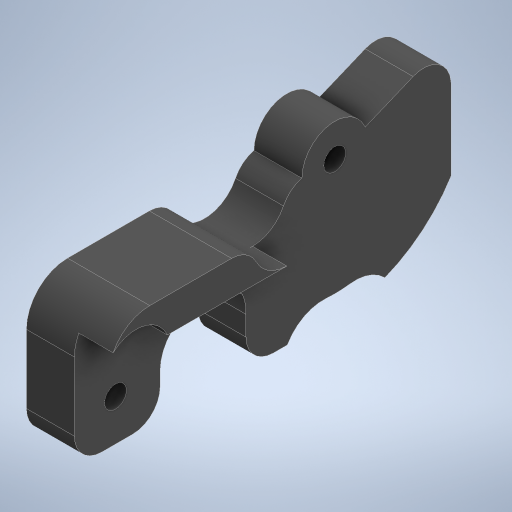
# Autodesk Inventor part: toe_springjoint_cover_under_right
Saved by Autodesk Inventor 2024.1 (Build 281209000, 209)
## iProperties
Created: 2024-02-25
Part Number: toe_springjoint_cover_under_right
Material: 一般
Document SubType Name: Modeling
Designer: hibik
Density: 1 g/cm^3
Appearance: 既定
Author: hibik
Autodesk Inventor part; units mm, degrees
ref_plane "YZ Plane" through (0, 0, 0) normal (1, 0, 0) x (0, 1, 0)
ref_plane "XZ Plane" through (0, 0, 0) normal (0, 1, 0) x (-1, 0, 0)
ref_plane "XY Plane" through (0, 0, 0) normal (0, 0, 1) x (1, 0, 0)
sketch "スケッチ1" plane through (0, 0, 0) normal (1, 0, 0) x (0, 1, 0)
  circle A0 centre (0, 0) radius 6 construction
  circle A1 centre (6, 0) radius 0.8
  line L0 (-14, 0) -> (14, 0)
  circle A2 centre (4.242641, 4.242641) radius 0.8
  circle A3 centre (0, 6) radius 0.8
  circle A4 centre (-4.242641, 4.242641) radius 0.8
  circle A5 centre (-6, 0) radius 0.8
  circle A6 centre (-4.242641, -4.242641) radius 0.8
  circle A7 centre (0, -6) radius 0.8
  circle A8 centre (4.242641, -4.242641) radius 0.8
  circle A9 centre (0, 0) radius 2.4
  line L1 (0, 0) -> (0, 6)
  line L2 (0, 0) -> (2.296101, -5.543277)
  circle A10 centre (0, 0) radius 10
  line L3 (2.296101, -5.543277) -> (3.826834, -9.238795)
  line L4 (0, -9.238795) -> (-10, -9.238795)
  line L5 (-10, -9.238795) -> (-10, 20)
  line L6 (-10, 20) -> (0, 20)
  line L7 (0, 20) -> (0, -9.238795)
  line L8 (0, -6) -> (4.242641, -4.242641) construction
  line L9 (0, -9.238795) -> (3.826834, -9.238795)
  circle A11 centre (0, 6) radius 2.5
  point P0 (0, 5.2)
  point P1 (0, 6.8)
  point P2 (-10, 0)
  point P3 (2.12132, -5.12132)
  point P4 (0, 2.4)
  point P5 (0.91844, -2.217311)
  point P6 (0, 8.5)
  point P7 (0, 10)
  point P8 (0, 3.5)
  point P9 (-3.826834, -9.238795)
  point P10 (0, -6.8)
  point P11 (0, -5.2)
  point P12 (0, -2.4)
  dimension "d1" = 12
  dimension "d2" = 1.6
  dimension "d5" = 360
  dimension "d7" = 4.8
  dimension "d8" = 4
  dimension "d21" = 5
  dimension "d23" = 20
  constraints: 18 end point, 11 centre point, 6 point on line, 5 coincident, 3 point on circle, 2 horizontal, 2 parallel, 1 midpoint, 1 perpendicular, 1 vertical, 20 other
  measures "d1" diameter of A0
  measures "d2" diameter of A1
  measures "d7" diameter of A9
  measures "d21" diameter of A11
  measures "d23" distance from line of L6 point (0, 0)
extrude "押し出し1" add sketch "スケッチ1" along normal blind 1.5 contours A9 L2 L0 | L0 L1 A9 | L9 L7 A7 A9 L2 L3 | L7 A11 L1 A9 L0 A5 A10 | A10 L5 L6 L7 | L7 A9 L0 | L0 A9 L1 | L2 A9 L7 | L4 L5 A10 | A10 L0 A5 A9 L7 A7 L4 | L7 A7 | A7 L7 | A5 L0 | L0 A5 | A4 | A6
sketch "スケッチ6" plane through (0, 0, 0) normal (-1, 0, 0) x (0, 0, 1)
  line L0 (12.746794, -7) -> (12.746794, -8)
  line L1 (17, -10) -> (14.746794, -10)
  line L2 (19, -8) -> (19, -3)
  arc A0 (19, -3) -> (16, 0) centre (16, -3) ccw
  line L3 (10.031129, 0) -> (16, 0)
  arc A1 (3.630208, 0.796296) -> (8.239516, -1.111111) centre (6, 0) ccw
  arc A2 (3.276042, 2.707407) -> (-3.926488, 1.626405) centre (0, 0) ccw
  line L4 (-5.713879, 2.366766) -> (-3.926488, 1.626405)
  arc A3 (-8.47286, 0.678702) -> (-8.5, 0) centre (0, 0) ccw
  line L5 (-8.5, 0) -> (-8.5, -5.267827)
  arc A4 (-8.5, -5.267827) -> (-3.6504, -9.309918) centre (0, 0) ccw
  arc A5 (-1.108696, -8.427384) -> (-3.6504, -9.309918) centre (-1.5, -11.401754) ccw
  arc A6 (-1.108696, -8.427384) -> (0.626747, -8.476862) centre (0, 0) ccw
  arc A7 (3.446028, -9.968696) -> (0.626747, -8.476862) centre (0.847952, -11.468696) ccw
  line L6 (3.446028, -9.968696) -> (3.464102, -10)
  line L7 (4.479657, -10) -> (3.464102, -10)
  line L8 (6.479657, -8) -> (6.479657, -6.559689)
  arc A8 (6.743932, -5.173913) -> (6.479657, -6.559689) centre (9.47607, -6.413035) ccw
  arc A9 (9.124144, -4) -> (6.743932, -5.173913) centre (9.124144, -7) ccw
  line L9 (9.124144, -4) -> (9.746794, -4)
  arc A10 (12.746794, -7) -> (9.746794, -4) centre (9.746794, -7) ccw
  circle A11 centre (17, -3.5) radius 0.8
  circle A12 centre (-6, 0) radius 0.8
  circle A13 centre (-4.242641, -4.242641) radius 0.8
  circle A14 centre (4.242641, -4.242641) radius 0.8
  circle A15 centre (0, -6) radius 0.8
  arc A16 (2.4, 0) -> (-2.217311, 0.91844) centre (0, 0) ccw
  line L10 (-9.238795, 3.826834) -> (-2.217311, 0.91844)
  line L11 (-9.238795, -10) -> (-9.238795, 3.826834)
  line L12 (20, -10) -> (-9.238795, -10)
  line L13 (20, 0) -> (20, -10)
  line L14 (8.5, 0) -> (20, 0)
  arc A17 (3.5, 0) -> (8.5, 0) centre (6, 0) ccw
  line L15 (2.4, 0) -> (3.5, 0)
  circle A18 centre (16, -7) radius 0.8
  circle A19 centre (0, 0) radius 0.8
  arc A20 (3.630208, 0.796296) -> (3.276042, 2.707407) centre (1.734375, 1.433333) ccw
  arc A21 (-5.713879, 2.366766) -> (-8.47286, 0.678702) centre (-6.479246, 0.519007) ccw
  arc A22 (4.479657, -10) -> (6.479657, -8) centre (4.479657, -8) ccw
  arc A23 (12.746794, -8) -> (14.746794, -10) centre (14.746794, -8) ccw
  arc A24 (17, -10) -> (19, -8) centre (17, -8) ccw
  arc A25 (10.031129, 0) -> (8.239516, -1.111111) centre (10.031129, -2) ccw
  point P0 (-7.852976, 3.252809)
  point P1 (6.479657, -10)
  point P2 (12.746794, -10)
  point P3 (16, 0)
  point P4 (19, -10)
  point P5 (-3.926488, 1.626405)
  point P6 (8.239516, -1.111111)
  point P7 (-3.926488, 1.626405)
  point P8 (16, 0)
extrude "押し出し5" cut sketch "スケッチ6" against normal through all contours L0 A23 L12 A22 L8 A8 A9 L9 A10 | A24 L2 A0 L14 L13 L12 | L12 L11 L10 A21 A3 L5 A4 A5 A6 A7 L6 | A25 A17 L14
sketch "スケッチ7" plane through (0, 0, 0) normal (-1, 0, 0) x (0, 0, 1)
  line L0 (14.5, -3.5) -> (6.629791, -3.5)
  arc A0 (-7.852976, 3.252809) -> (-8.5, 0) centre (0, 0) ccw
  line L1 (-8.5, 0) -> (-8.5, -5.267827)
  arc A1 (-8.5, -5.267827) -> (-3.6504, -9.309918) centre (0, 0) ccw
  arc A2 (-1.108696, -8.427384) -> (-3.6504, -9.309918) centre (-1.5, -11.401754) ccw
  arc A3 (-1.108696, -8.427384) -> (0.626747, -8.476862) centre (0, 0) ccw
  arc A4 (3.446028, -9.968696) -> (0.626747, -8.476862) centre (0.847952, -11.468696) ccw
  line L2 (3.446028, -9.968696) -> (3.464102, -10)
  line L3 (6.479657, -10) -> (3.464102, -10)
  line L4 (6.479657, -10) -> (6.479657, -6.559689)
  arc A5 (6.743932, -5.173913) -> (6.479657, -6.559689) centre (9.47607, -6.413035) ccw
  arc A6 (9.124144, -4) -> (6.743932, -5.173913) centre (9.124144, -7) ccw
  line L5 (9.124144, -4) -> (9.746794, -4)
  arc A7 (12.746794, -7) -> (9.746794, -4) centre (9.746794, -7) ccw
  line L6 (12.746794, -7) -> (12.746794, -10)
  line L7 (19, -10) -> (12.746794, -10)
  line L8 (19, -10) -> (19, -3)
  arc A8 (19, -3) -> (16, 0) centre (16, -3) ccw
  line L9 (8.5, 0) -> (16, 0)
  arc A9 (3.5, 0) -> (8.5, 0) centre (6, 0) ccw
  line L10 (2.4, 0) -> (3.5, 0)
  arc A10 (2.4, 0) -> (-2.217311, 0.91844) centre (0, 0) ccw
  line L11 (-7.852976, 3.252809) -> (-2.217311, 0.91844)
  circle A11 centre (17, -3.5) radius 0.8
  circle A12 centre (17, -3.5) radius 2.5
  line L12 (6.629791, -3.5) -> (0, -3.5)
  circle A13 centre (0, 0) radius 3.5
  line L13 (3.5, 0) -> (3.5, -3.5)
  line L14 (0, -3.5) -> (14.708712, -3.5)
  line L15 (14.708712, -3.5) -> (14.708712, -2.5)
  line L16 (14.708712, -2.5) -> (0, -2.5)
  line L17 (0, -2.5) -> (0, -3.5)
  point P0 (18.677033, -1.645934)
  point P1 (6, -2.5)
  dimension "d31" = 5
  dimension "d34" = 1
  constraints: 12 end point, 3 horizontal, 2 coincident, 2 parallel, 2 perpendicular, 1 collinear, 1 point on line, 1 tangent, 1 vertical, 1 vertical alignment, 5 other
  measures "d34" distance between parallel lines of L16 L0
extrude "押し出し6" add sketch "スケッチ7" along normal blind 2.5 contours L16 A9 L9 A8 A12
sketch "スケッチ8" plane through (1.5, 0, 0) normal (1, 0, 0) x (0, 0, -1)
  circle A0 centre (-16, -7) radius 0.8
  line L0 (-17, -10) -> (-14.746794, -10)
  line L1 (-19, -3) -> (-19, -8)
  circle A1 centre (0, 0) radius 0.8
  point P0 (-19, -10)
  point P1 (-12.746794, -10)
  dimension "d35" = 1.6
  dimension "d36" = 3
  dimension "d37" = 3
  dimension "d40" = 1.6
  constraints: 2 centre point, 1 coincident
  measures "d35" diameter of A0
  measures "d36" distance from line of L0 A0.centre
  measures "d37" distance from line of L1 A0.centre
  measures "d40" diameter of A1
extrude "押し出し7" cut sketch "スケッチ8" against normal through all
fillet "フィレット1" radius 2 2 edges at (0.75, 0, 3.5) (-1.25, 0, 8.5)
sketch "スケッチ9" plane through (0, 0, 0) normal (-1, 0, 0) x (0, 0, 1)
  arc A0 (3.74614, -1.08172) -> (2.4, 0) centre (1.943053, -1.947095) ccw
  arc A1 (2.4, 0) -> (-2.217311, 0.91844) centre (0, 0) ccw
  line L0 (-5.713879, 2.366766) -> (-2.217311, 0.91844)
  arc A2 (-5.713879, 2.366766) -> (-8.47286, 0.678702) centre (-6.479246, 0.519007) ccw
  arc A3 (-8.47286, 0.678702) -> (-8.5, 0) centre (0, 0) ccw
  line L1 (-8.5, 0) -> (-8.5, -5.267827)
  arc A4 (-8.5, -5.267827) -> (-3.6504, -9.309918) centre (0, 0) ccw
  arc A5 (-1.108696, -8.427384) -> (-3.6504, -9.309918) centre (-1.5, -11.401754) ccw
  arc A6 (-1.108696, -8.427384) -> (0.626747, -8.476862) centre (0, 0) ccw
  arc A7 (3.446028, -9.968696) -> (0.626747, -8.476862) centre (0.847952, -11.468696) ccw
  line L2 (3.446028, -9.968696) -> (3.464102, -10)
  line L3 (4.479657, -10) -> (3.464102, -10)
  arc A8 (4.479657, -10) -> (6.479657, -8) centre (4.479657, -8) ccw
  line L4 (6.479657, -8) -> (6.479657, -6.559689)
  arc A9 (6.743932, -5.173913) -> (6.479657, -6.559689) centre (9.47607, -6.413035) ccw
  arc A10 (9.124144, -4) -> (6.743932, -5.173913) centre (9.124144, -7) ccw
  line L5 (9.124144, -4) -> (9.746794, -4)
  arc A11 (12.746794, -7) -> (9.746794, -4) centre (9.746794, -7) ccw
  line L6 (12.746794, -7) -> (12.746794, -8)
  arc A12 (12.746794, -8) -> (14.746794, -10) centre (14.746794, -8) ccw
  line L7 (17, -10) -> (14.746794, -10)
  arc A13 (17, -10) -> (19, -8) centre (17, -8) ccw
  line L8 (19, -8) -> (19, -3)
  arc A14 (19, -3) -> (18.677033, -1.645934) centre (16, -3) ccw
  arc A15 (18.677033, -1.645934) -> (14.708712, -2.5) centre (17, -3.5) ccw
  line L9 (14.708712, -2.5) -> (6, -2.5)
  arc A16 (3.74614, -1.08172) -> (6, -2.5) centre (6, 0) ccw
  circle A17 centre (16, -7) radius 0.8
  circle A18 centre (0, 0) radius 0.8
extrude "押し出し8" add sketch "スケッチ9" along normal blind 2
sketch "スケッチ10" plane through (-2.5, 0, 0) normal (-1, 0, 0) x (0, 0, 1)
  arc A0 (10.031129, 0) -> (8.239516, -1.111111) centre (10.031129, -2) ccw
  arc A1 (6, -2.5) -> (8.239516, -1.111111) centre (6, 0) ccw
  line L0 (6, -2.5) -> (14.708712, -2.5)
  arc A2 (18.677033, -1.645934) -> (14.708712, -2.5) centre (17, -3.5) ccw
  arc A3 (18.677033, -1.645934) -> (16, 0) centre (16, -3) ccw
  line L1 (16, 0) -> (10.031129, 0)
  point P0 (0, 0)
extrude "押し出し9" add sketch "スケッチ10" along normal blind 2
mirror "ミラー1" about plane through (0, 0, 0) normal (1, 0, 0) remove original yes
